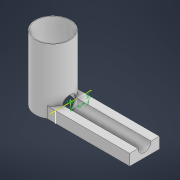
# Autodesk Inventor part: 直線軌道
Saved by Autodesk Inventor 2021 (Build 250183000, 183)
## iProperties
Created: 2020-12-30
Part Number: 直線軌道
Material: 一般
Document SubType Name: Modeling
Designer: zihon
Density: 1 g/cm^3
Appearance: 預設
Author: zihon
Autodesk Inventor part; units mm, degrees
ref_plane "YZ Plane" through (0, 0, 0) normal (1, 0, 0) x (0, 1, 0)
ref_plane "XZ Plane" through (0, 0, 0) normal (0, 1, 0) x (-1, 0, 0)
ref_plane "XY Plane" through (0, 0, 0) normal (0, 0, 1) x (1, 0, 0)
sketch "草圖1" plane through (0, 0, 0) normal (1, 0, 0) x (0, 1, 0)
  arc A0 (0, 17.5) -> (0, -17.5) centre (0, 0) ccw
  arc A1 (0, 20) -> (0, -20) centre (0, 0) ccw
  line L0 (0, 17.5) -> (0, 20)
  line L1 (0, -20) -> (0, -17.5)
  line L2 (0, -56) -> (0, 56) projected
  line L3 (0, -40) -> (-30, -40)
  line L4 (-30, -40) -> (-30, -20)
  line L5 (0, -40) -> (0, -20)
  line L6 (-36, 0) -> (6, 0) projected
  line L7 (0, 40) -> (-30, 40)
  line L8 (-30, 40) -> (-30, -20)
  point P0 (0, -20)
  dimension "d0" = 17.5
  dimension "d1" = 20
  dimension "d4" = 30
  dimension "d5" = 40
  constraints: 14 end point, 4 point on circle, 3 collinear, 2 centre point, 2 coincident, 2 vertical, 2 vertical alignment, 1 horizontal, 1 perpendicular, 1 point on line, 1 other
  measures "d0" radius of A0
  measures "d1" radius of A1
  measures "d4" distance of L3.start L3.end
  measures "d5" distance of the line from the sketch origin of L3
extrude "擠出1" add sketch "草圖1" along normal blind 200 contours A0 L6 A1 L0 | A0 L1 A1 L6 | A1 L6 L8 L7 L2 | A1 L2 L3 L4 L8 L6
sketch "草圖3" plane through (0, -30, -40) normal (0, -1, 0) x (1, 0, 0)
  circle A0 centre (-47.101, 40) radius 45.101
  circle A1 centre (-47.101, 40) radius 47.101
  line L0 (-153.0424, 40) -> (258.8404, 40) projected
  line L1 (0, 80) -> (0, 0) projected
  point P0 (0, 40)
  dimension "d6" = 90.202
  dimension "d7" = 2
  constraints: 2 centre point, 1 point on line, 1 tangent
  measures "d6" diameter of A0
  measures "d7" radial gap between concentric circles of A0 A1
extrude "擠出2" add sketch "草圖3" against normal blind 175 contours L0 A1 A0 | A0 L0 A1
extrude "擠出3" add sketch "草圖1" against normal up to surface contours A0 L6 A1 L0 | A0 L1 A1 L6 | A1 L6 L8 L7 L2 | A1 L2 L3 L4 L8 L6
sketch "草圖4" plane through (200, 0, 0) normal (1, 0, 0) x (0, 0, -1)
  arc A0 (-17.5, 0) -> (17.5, 0) centre (0, 0) ccw projected
  circle A1 centre (0, 0) radius 17.5
  constraints: 1 coincident, 3 other
extrude "擠出4" cut sketch "草圖4" against normal up to surface
